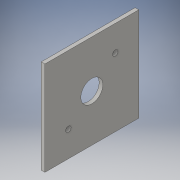
# Autodesk Inventor part: Guard Plate
Saved by Autodesk Inventor 2016 SP2 (Build 200236200, 236)
## iProperties
Created: 2018-01-13
Part Number: Guard Plate
Material: Generic
Document SubType Name: Modeling
Designer: CAD
Density: 1 g/cm^3
Appearance: Default
Author: CAD
Autodesk Inventor part; units mm, degrees
ref_plane "YZ Plane" through (0, 0, 0) normal (1, 0, 0) x (0, 1, 0)
ref_plane "XZ Plane" through (0, 0, 0) normal (0, 1, 0) x (-1, 0, 0)
ref_plane "XY Plane" through (0, 0, 0) normal (0, 0, 1) x (1, 0, 0)
sketch "Sketch1" plane through (0, 0, 0) normal (1, 0, 0) x (0, 1, 0)
  line L0 (11.2555, 71.2167) -> (-70.0245, 71.2167)
  line L1 (-70.0245, 71.2167) -> (-70.0245, -10.0633)
  line L2 (-70.0245, -10.0633) -> (11.2555, -10.0633)
  line L3 (11.2555, -10.0633) -> (11.2555, 71.2167)
  point P0 (0, 0)
  dimension "d0" = 81.28
  dimension "d1" = 81.28
  constraints: 8 end point, 2 parallel, 1 horizontal, 1 perpendicular
  measures "d0" distance of L2.end L1.end
  measures "d1" distance of L2.end L0.start
extrude "Extrusion1" add sketch "Sketch1" along normal blind 3.175
sketch "Sketch2" plane through (3.175, 0, 0) normal (1, 0, 0) x (0, 0, -1)
  circle A0 centre (-30.5767, -29.3845) radius 9.525
  line L0 (10.0633, 11.2555) -> (-71.2167, 11.2555) projected
  line L1 (-71.2167, 11.2555) -> (-71.2167, -70.0245) projected
  circle A1 centre (-10.2567, -10.9695) radius 2.3495
  circle A2 centre (-50.8967, -47.7995) radius 2.3495
  line L2 (-71.2167, -70.0245) -> (10.0633, -70.0245) projected
  line L3 (10.0633, -70.0245) -> (10.0633, 11.2555) projected
  point P0 (0, 0)
  dimension "d4" = 19.05
  dimension "d5" = 40.64
  dimension "d6" = 40.64
  dimension "d9" = 4.699
  dimension "d10" = 4.699
  dimension "d11" = 20.32
  dimension "d12" = 22.225
  dimension "d13" = 22.225
  dimension "d14" = 20.32
  constraints: 3 centre point
  measures "d4" diameter of A0
  measures "d5" distance from line of L0 A0.centre
  measures "d6" distance from line of A0.centre L1
  measures "d9" diameter of A1
  measures "d10" diameter of A2
  measures "d11" distance from line of L1 A2.centre
  measures "d12" distance from line of L2 A2.centre
  measures "d13" distance from line of L0 A1.centre
  measures "d14" distance from line of L3 A1.centre
extrude "Extrusion2" cut sketch "Sketch2" against normal blind 3.175 contours A0 | A1 | A2
body "Solid1"
